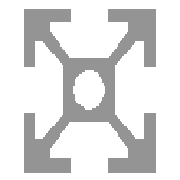
# Autodesk Inventor part: 20x20 Channel-860
Saved by Autodesk Inventor 2023 (Build 270158000, 158)
## iProperties
Created: 2022-07-10
Part Number: 20x20 Channel-860
Material: Aluminum 6061
Document SubType Name: Modeling
Designer: DavidK
Density: 2.7 g/cm^3
Appearance: Aluminum - Flat
Categories: <MemberInstance><Categories><Category DisplayName="Structural Shapes" InternalName="089c4875-fa83-4c05-b084-43b9cc11f5ed" Mnemonic="GRDR"><CategoryParameter DisplayName="Mass per Length Unit" InternalName="0bb95a10-148f-4027-a459-38d7b056702a" Mnemonic="shpmass"/><CategoryParameter DisplayName="Section Area" InternalName="1ff91680-64b0-4202-b9a3-7fd3f94bba3b" Mnemonic="secarea"/><CategoryParameter DisplayName="Radius of Gyration (x)" InternalName="25778675-03e9-40c1-b6a8-4a9ed693320d" Mnemonic="gyrradx"/><CategoryParameter DisplayName="Torsional Rigidity Modulus" InternalName="26c1ec35-5026-4c63-ad0a-751cf684a536" Mnemonic="torrigmod"/><CategoryParameter DisplayName="Distance of the Center of Gravity X-X" InternalName="26c9bdb8-9c79-4b4f-a92e-8e197583c9c4" Mnemonic="grcendistX"/><CategoryParameter DisplayName="Legacy Member ID" InternalName="340afe4f-75d7-48d3-ab7d-943f3c3da468" Mnemonic="LegacyMemberID"/><CategoryParameter DisplayName="Base Length" InternalName="42e34263-8f20-4d0e-ad48-bf1385b87c24" Mnemonic="shplen"/><CategoryParameter DisplayName="Moment of Inertia (y)" InternalName="4b9f58ea-bced-460e-81ea-3d29ca5a49e3" Mnemonic="inermomy"/><CategoryParameter DisplayName="Moment of Inertia (x)" InternalName="4cd780bc-73d7-43ac-917a-579e5cbd684d" Mnemonic="inermomx"/><CategoryParameter DisplayName="Custom Base Point" InternalName="4f1d1b73-316d-484b-a3df-9cbabb16eb77" Mnemonic="shpBasePoint"/><CategoryParameter DisplayName="Shape Height" InternalName="50274e7d-5ac0-4796-92cb-c59e54983c67" Mnemonic="shpheig"/><CategoryParameter DisplayName="Section Module (y)" InternalName="59eaa5e9-d227-48dc-b6c1-6920f96e0f95" Mnemonic="secmody"/><CategoryParameter DisplayName="Section Designation" InternalName="5a64d034-428d-49c8-ba32-7619764de20f" Mnemonic="shpdes"/><CategoryParameter DisplayName="Section Module (x)" InternalName="72cfad18-cf51-4ed4-aaa7-c6b224f8419f" Mnemonic="secmodx"/><CategoryParameter DisplayName="Torsional Section Modulus" InternalName="7c55a8dc-8844-49f9-a867-cc677b30ec9a" Mnemonic="torsecmod"/><CategoryParameter DisplayName="Shape Width" InternalName="7c717d54-a18f-4666-b4d4-573cce22c62c" Mnemonic="shpwdth"/><CategoryParameter DisplayName="Second Shape Thickness" InternalName="9251a8e1-85fd-4e47-af99-afdb762317d9" Mnemonic="shpthick2"/><CategoryParameter DisplayName="FG Authored" InternalName="9c666724-f362-4ea7-ac62-f6a007de5c69" Mnemonic="shpFGAuto"/><CategoryParameter DisplayName="Distance of the Center of Gravity Y-Y" InternalName="bcc4fb17-7af4-436a-8f8c-d0aa3b0248c5" Mnemonic="grcendistY"/><CategoryParameter DisplayName="Radius of Gyration (y)" InternalName="bfa18ebe-1636-4dbe-8d42-b263e0b73184" Mnemonic="gyrrady"/><CategoryParameter DisplayName="Shape Thickness" InternalName="d109cf76-8eb4-42fc-9800-4409734adc67" Mnemonic="shpthick"/><CategoryParameter DisplayName="Coefficient of Shear Displacement" InternalName="de4c90c6-aaa8-468f-a335-6737b311b5d3" Mnemonic="shdispc"/><Category DisplayName="Other" InternalName="f02205ff-2390-476f-921c-0b3185f88e84" Mnemonic="OTHSHP"><CategoryParameter DisplayName="Moment of Inertia (y)" InternalName="044c654e-f649-48ac-84cc-650a29ae31ca" Mnemonic="inermomy"/><CategoryParameter DisplayName="Shape Thickness" InternalName="12b1a788-9233-48fd-a933-2df8ff42b15f" Mnemonic="shpthick"/><CategoryParameter DisplayName="Mass per Length Unit" InternalName="2fd289d6-9394-4d2d-97e6-6659d7d4551d" Mnemonic="shpmass"/><CategoryParameter DisplayName="Radius of Gyration (y)" InternalName="743e1dfe-1bba-408b-b985-cf752b207386" Mnemonic="gyrrady"/><CategoryParameter DisplayName="Section Module (y)" InternalName="88b8bff9-a616-4028-93d5-ed4f79680d13" Mnemonic="secmody"/><CategoryParameter DisplayName="Section Area" InternalName="c46ecdf8-b6eb-4db9-8b25-30258930c1e3" Mnemonic="secarea"/><CategoryParameter DisplayName="Section Module (x)" InternalName="cac70804-9d39-43bb-be17-56ea1f39a6c2" Mnemonic="secmodx"/><CategoryParameter DisplayName="Moment of Inertia (x)" InternalName="ec6737bc-264f-43ed-b0bd-f6d410c2718d" Mnemonic="inermomx"/><CategoryParameter DisplayName="Radius of Gyration (x)" InternalName="ee72c61e-565e-4fd6-b448-66e1e1abcb7e" Mnemonic="gyrradx"/></Category></Category></Categories><FamilyTemplate Id="20x20 Channel"><FamilyTemplateParameters><FamilyTemplateParameter ObjectType="kModelParameterObject" ValueType="xs:double" Id="12" ObjectReferenceKey="ChannelLength"/></FamilyTemplateParameters></FamilyTemplate><CategoryParameterMap><ParamToTemplateMap><ParamToTemplate CategoryParameter="//CategoryParameter[@InternalName='9c666724-f362-4ea7-ac62-f6a007de5c69']" ConstantValue="1"/><ParamToTemplate CategoryParameter="//CategoryParameter[@InternalName='42e34263-8f20-4d0e-ad48-bf1385b87c24']" TemplateParameter="12"/></ParamToTemplateMap></CategoryParameterMap></MemberInstance>
Mass: 209.727 g
Surface Area: 849.96 cm^2
Volume: 77.6765 cm^3
Length: 860.000 mm
Author: Dave
Autodesk Inventor part; units mm, degrees
ref_plane "YZ Plane" through (0, 0, 0) normal (1, 0, 0) x (0, 1, 0)
ref_plane "XZ Plane" through (0, 0, 0) normal (0, 1, 0) x (-1, 0, 0)
ref_plane "XY Plane" through (0, 0, 0) normal (0, 0, 1) x (1, 0, 0)
sketch "Sketch2" plane through (0, 0, 0) normal (1, 0, 0) x (0, 1, 0)
  line L0 (1, 0) -> (19, 0)
  line L1 (20, -1) -> (20, -19)
  line L2 (19, -20) -> (1, -20)
  line L3 (0, -19) -> (0, -1)
  circle A0 centre (10, -10) radius 2.5
  line L4 (13.9, -6.1) -> (6.1, -6.1)
  line L5 (6.1, -6.1) -> (6.1, -13.9)
  line L6 (6.1, -13.9) -> (13.9, -13.9)
  line L7 (13.9, -13.9) -> (13.9, -6.1)
  line L8 (13.1, -20) -> (13.1, -18.6)
  line L9 (13.1, -18.6) -> (16.2101, -18.6)
  line L10 (16.2101, -18.6) -> (16.2101, -17.2)
  line L11 (16.2101, -17.2) -> (12.9101, -13.9)
  line L12 (10, -20) -> (10, -13.9) construction
  line L13 (6.9, -18.6) -> (3.7899, -18.6)
  line L14 (3.7899, -18.6) -> (3.7899, -17.2)
  line L15 (3.7899, -17.2) -> (7.0899, -13.9)
  line L16 (6.9, -18.6) -> (6.9, -20)
  line L17 (1.4, -6.9) -> (1.4, -3.7899)
  line L18 (1.4, -6.9) -> (0, -6.9)
  line L19 (1.4, -3.7899) -> (2.8, -3.7899)
  line L20 (2.8, -3.7899) -> (6.1, -7.0899)
  line L21 (0, -13.1) -> (1.4, -13.1)
  line L22 (1.4, -13.1) -> (1.4, -16.2101)
  line L23 (1.4, -16.2101) -> (2.8, -16.2101)
  line L24 (2.8, -16.2101) -> (6.1, -12.9101)
  line L25 (13.1, -1.4) -> (16.2101, -1.4)
  line L26 (13.1, -1.4) -> (13.1, 0)
  line L27 (16.2101, -1.4) -> (16.2101, -2.8)
  line L28 (16.2101, -2.8) -> (12.9101, -6.1)
  line L29 (6.9, 0) -> (6.9, -1.4)
  line L30 (6.9, -1.4) -> (3.7899, -1.4)
  line L31 (3.7899, -1.4) -> (3.7899, -2.8)
  line L32 (3.7899, -2.8) -> (7.0899, -6.1)
  line L33 (18.6, -13.1) -> (18.6, -16.2101)
  line L34 (18.6, -13.1) -> (20, -13.1)
  line L35 (18.6, -16.2101) -> (17.2, -16.2101)
  line L36 (17.2, -16.2101) -> (13.9, -12.9101)
  line L37 (20, -6.9) -> (18.6, -6.9)
  line L38 (18.6, -6.9) -> (18.6, -3.7899)
  line L39 (18.6, -3.7899) -> (17.2, -3.7899)
  line L40 (17.2, -3.7899) -> (13.9, -7.0899)
  arc A1 (20, -1) -> (19, 0) centre (19, -1) ccw
  arc A2 (19, -20) -> (20, -19) centre (19, -19) ccw
  arc A3 (0, -19) -> (1, -20) centre (1, -19) ccw
  arc A4 (1, 0) -> (0, -1) centre (1, -1) ccw
  point P0 (0, 0)
  point P1 (20, -20)
  point P2 (20, 0)
  point P3 (0, -20)
  point P4 (20, -10)
  point P5 (13.9, -10)
  point P6 (14.655, -18.6)
  point P7 (1.4, -14.655)
  point P8 (5.345, -1.4)
  point P9 (18.6, -5.345)
  point P10 (13.9, -12.9101)
  point P11 (13.9, -7.0899)
  point P12 (20, -6.9)
  point P13 (13.1, 0)
  point P14 (12.9101, -6.1)
  point P15 (7.0899, -6.1)
  point P16 (6.9, 0)
  point P17 (0, -6.9)
  point P18 (6.1, -7.0899)
  point P19 (6.1, -12.9101)
  point P20 (0, -13.1)
  point P21 (20, -13.1)
  dimension "d0" = 20
  dimension "d1" = 20
  dimension "d2" = 5
  dimension "d3" = 6.1
  dimension "d4" = 6.1
  dimension "d5" = 6.2
  dimension "d6" = 1.4
  dimension "d7" = 0.7
  dimension "d8" = 45
  dimension "d9" = 1.4
  dimension "d12" = 360
  dimension "d29" = 1
  constraints: 82 end point, 12 point on line, 8 point on circle, 8 tangent, 5 centre point, 5 midpoint, 5 perpendicular, 4 parallel, 3 equal radius, 3 symmetric about line, 2 coincident, 2 horizontal, 2 horizontal alignment, 2 vertical, 2 vertical alignment, 80 other
  measures "d0" distance of point (20, -20) point (0, -20)
  measures "d1" distance of point (20, 0) point (20, -20)
  measures "d2" diameter of A0
  measures "d3" distance between parallel lines of L2 L6
  measures "d4" distance between parallel lines of L1 L7
  measures "d5" distance between parallel lines of L16 L8
  measures "d6" distance from line of L2 point (14.655, -18.6)
  measures "d7" distance from line of L6.end L11
  measures "d8" angle of L11 L6
  measures "d9" distance of L9.end L10.end
  measures "d29" radius of A1
extrude "Extrusion3" add sketch "Sketch2" along normal blind 860 contours L0 L29 L30 L31 L32 L4 L5 L20 L19 L17 L18 L3 A4 | L0 A1 L1 L37 L38 L39 L40 L7 L4 L28 L27 L25 L26 | L21 L22 L23 L24 L5 L6 L15 L14 L13 L16 L2 A3 L3 | L4 L7 L6 L5 | L1 A2 L2 L8 L9 L10 L11 L6 L7 L36 L35 L33 L34
fillet "Fillet2" radius 1 32 edges at (430, 17.2, -16.2101) (430, 18.6, -16.2101) (430, 20, -13.1) (430, 20, -6.9) (430, 18.6, -3.7899) (430, 17.2, -3.7899) (430, 13.9, -7.0899) (430, 13.9, -12.9101) (430, 13.1, -20) (430, 16.2101, -18.6) (430, 16.2101, -17.2) (430, 12.9101, -13.9) (430, 7.0899, -13.9) (430, 3.7899, -17.2) (430, 3.7899, -18.6) (430, 6.9, -20) (430, 0, -13.1) (430, 1.4, -16.2101) (430, 2.8, -16.2101) (430, 6.1, -12.9101) (430, 6.1, -7.0899) (430, 2.8, -3.7899) (430, 1.4, -3.7899) (430, 0, -6.9) (430, 3.7899, -2.8) (430, 3.7899, -1.4) (430, 6.9, 0) (430, 7.0899, -6.1) (430, 13.1, 0) (430, 16.2101, -1.4) (430, 16.2101, -2.8) (430, 12.9101, -6.1)
equation "\"d7\" = 0.5 * d6"
equation "\"d9\" = d6"
equation "\"d27\" = Length"
equation "\"Length\" = 860"
body "Solid2"
